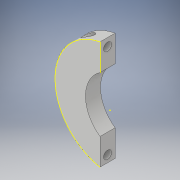
# Autodesk Inventor part: Contrapeso5
Saved by Autodesk Inventor 2019.3 (Build 233278000, 278)
## iProperties
Created: 2019-06-29
Part Number: Contrapeso5
Material: Generic
Document SubType Name: Modeling
Designer: usuario
Density: 1 g/cm^3
Appearance: Default
Mass: 5.56788 g
Surface Area: 27.2211 cm^2
Volume: 5.56788 cm^3
Author: usuario
Autodesk Inventor part; units mm, degrees
ref_plane "YZ Plane" through (0, 0, 0) normal (1, 0, 0) x (0, 1, 0)
ref_plane "XZ Plane" through (0, 0, 0) normal (0, 1, 0) x (-1, 0, 0)
ref_plane "XY Plane" through (0, 0, 0) normal (0, 0, 1) x (1, 0, 0)
sketch "Sketch1" plane through (0, 0, 0) normal (0, 0, 1) x (1, 0, 0)
  arc A0 (0, 27.5) -> (0, -27.5) centre (0, 0) ccw
  arc A1 (-5, 13.7954) -> (-5, -13.7954) centre (4.5, 0) ccw
  line L0 (-5, -27.0416) -> (-5, -13.7954)
  arc A2 (-5, 27.0416) -> (-5, -27.0416) centre (0, 0) ccw
  line L1 (-5, 27.0416) -> (-5, 13.7954)
  point P0 (3.7885, 24.6247)
  point P1 (-3.7885, 24.6247)
  point P2 (-4.5, 0)
  point P3 (5, 27.5)
  constraints: 6 point on circle, 4 end point, 3 centre point, 1 coincident
extrude "Extrusion1" add sketch "Sketch1" along normal blind 7.5
sketch "Sketch2" plane through (-5, -27.0416, 0) normal (1, 0, 0) x (0, 0, -1)
  line L0 (0, 6.9167) -> (7.5, 6.9167)
  line L1 (0, 0) -> (0, 6.9167)
  line L2 (0, 6.9167) -> (7.5, 6.9167)
  line L3 (7.5, 26.7893) -> (7.5, 0)
  line L4 (7.5, 6.9167) -> (7.5, 0)
  line L5 (7.5, 0) -> (0, 0)
  line L6 (7.5, 0) -> (0, 0)
  circle A0 centre (3.75, 3.4583) radius 1
  line L7 (0, 0) -> (3.0149, 2.7804)
  line L8 (4.4851, 4.1363) -> (7.5, 6.9167)
  line L9 (0, 6.9167) -> (3.0149, 4.1363)
  line L10 (4.4851, 2.7804) -> (7.5, 0)
  line L11 (0, 0) -> (0, 53.5786)
  line L12 (0, 53.5786) -> (0, 0)
  line L13 (0, 26.7893) -> (7.5, 26.7893)
  circle A1 centre (3.75, 50.1203) radius 1
  circle A2 centre (-3.75, 3.4583) radius 1
  circle A3 centre (-3.75, 50.1203) radius 1
  circle A4 centre (-3.75, 3.4583) radius 2
  circle A5 centre (-3.75, 50.1203) radius 2
  point P0 (0, 27.0416)
  point P1 (280.32, 51.414)
  dimension "d2" = 2
  dimension "d5" = 4
  dimension "d6" = 4
  constraints: 28 end point, 6 centre point, 4 point on circle, 3 symmetric about line, 2 coincident, 2 perpendicular, 2 vertical, 1 collinear, 1 midpoint, 3 other
  measures "d2" diameter of A0
  measures "d5" diameter of A4
  measures "d6" diameter of A5
extrude "Extrusion2" cut sketch "Sketch2" against normal blind 25.4 contours A2 | A3
extrude "Extrusion3" cut sketch "Sketch2" against normal blind 18.575 contours A2 | A3 | A4 | A5
sketch "Sketch3" plane through (0, 0, 7.5) normal (0, 0, 1) x (1, 0, 0)
  line L0 (-5, 13.7954) -> (-5, 27.0416) projected
  arc A0 (-5, 27.0416) -> (-5, -27.0416) centre (0, 0) ccw projected
  constraints: 1 point on circle
body "Solid1"
